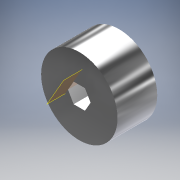
# Autodesk Inventor part: Pulley
Saved by Autodesk Inventor 2019.4 (Build 234330000, 330)
## iProperties
Created: 2020-01-24
Part Number: Pulley
Material: Aluminum 6061
Document SubType Name: Modeling
Designer: Mark
Mass: 164.314 g
Surface Area: 267.901 cm^2
Volume: 60.857 cm^3
Density: 2.7 g/cm^3
Appearance: Aluminum - Flat
Author: Mark
Autodesk Inventor part; units mm, degrees
ref_plane "YZ Plane" through (0, 0, 0) normal (1, 0, 0) x (0, 1, 0)
ref_plane "XZ Plane" through (0, 0, 0) normal (0, 1, 0) x (-1, 0, 0)
ref_plane "XY Plane" through (0, 0, 0) normal (0, 0, 1) x (1, 0, 0)
sketch "Sketch1" plane through (0, 0, 0) normal (0, 0, 1) x (1, 0, 0)
  circle A0 centre (0, 0) radius 25
  line L0 (3.695, 6.4) -> (7.3901, 0)
  line L1 (7.3901, 0) -> (3.695, -6.4)
  line L2 (3.695, -6.4) -> (-3.695, -6.4)
  line L3 (-3.695, -6.4) -> (-7.3901, 0)
  line L4 (-7.3901, 0) -> (-3.695, 6.4)
  line L5 (-3.695, 6.4) -> (3.695, 6.4)
  line L6 (0, 0) -> (0, -6.4) construction
  line L7 (0, 0) -> (6.4, 0) construction
  dimension "d0" = 50
  dimension "d1" = 12.8
  dimension "d2" = 90
  dimension "d3" = 90
  constraints: 16 end point, 2 coincident, 1 centre point, 1 horizontal, 1 midpoint, 1 perpendicular, 13 other
  measures "d0" diameter of A0
  measures "d1" distance between parallel lines of L2 L5
  measures "d2" angle of L6 L7
  measures "d3" angle of L2 L6
extrude "Extrusion1" add sketch "Sketch1" along normal blind 26
ref_plane "Work Plane1" through (-3.695, 6.4, 27) normal (0.8660254, -0.5, 0) x (0, 0, -1)
sketch "Sketch4" plane through (-3.695, 6.4, 27) normal (0.8660254, -0.5, 0) x (0, 0, -1)
  circle A0 centre (14, -3.695) radius 2.5
  line L0 (27, -28.695) -> (27, 21.305) projected
  line L1 (27, 0) -> (1, 0) projected
  dimension "d12" = 5
  dimension "d19" = 13
  dimension "d20" = 3.695
  constraints: 1 centre point
  measures "d12" diameter of A0
  measures "d19" distance from line of L0 A0.centre
  measures "d20" distance from line of L1 A0.centre
extrude "Extrusion4" cut sketch "Sketch4" against normal up to surface round surface about axis through (0, 0, 0) along (0, 0, 1) radius 25 far side no
body "Solid1"
